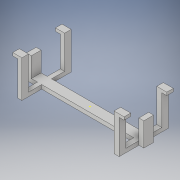
# Autodesk Inventor part: BatteryHanger
Saved by Autodesk Inventor 2018.2 (Build 222227000, 227)
## iProperties
Created: 2018-03-31
Part Number: BatteryHanger
Material: Generic
Document SubType Name: Modeling
Designer: MIABo
Density: 1 g/cm^3
Appearance: Default
Author: MIABo
Autodesk Inventor part; units mm, degrees
ref_plane "YZ Plane" through (0, 0, 0) normal (1, 0, 0) x (0, 1, 0)
ref_plane "XZ Plane" through (0, 0, 0) normal (0, 1, 0) x (-1, 0, 0)
ref_plane "XY Plane" through (0, 0, 0) normal (0, 0, 1) x (1, 0, 0)
sketch "Sketch1" plane through (0, 0, 0) normal (0, 1, 0) x (-1, 0, 0)
  line L0 (69.3801, 23.2918) -> (-69.3801, 23.2918)
  line L1 (-69.3801, 23.2918) -> (-69.3801, -23.2918)
  line L2 (-69.3801, -23.2918) -> (69.3801, -23.2918)
  line L3 (69.3801, -23.2918) -> (69.3801, 23.2918)
  line L4 (69.3801, 23.2918) -> (-69.3801, -23.2918) construction
  line L5 (-69.3801, 23.2918) -> (69.3801, -23.2918) construction
  line L6 (69.3801, -6.35) -> (-69.3801, -6.35)
  line L7 (-69.3801, -6.35) -> (-69.3801, 6.35)
  line L8 (-69.3801, 6.35) -> (69.3801, 6.35)
  line L9 (69.3801, 6.35) -> (69.3801, -6.35)
  line L10 (69.3801, -6.35) -> (-69.3801, 6.35) construction
  line L11 (-69.3801, -6.35) -> (69.3801, 6.35) construction
  line L12 (-62.7307, -31.75) -> (-69.3801, -31.75)
  line L13 (-69.3801, -31.75) -> (-69.3801, 31.75)
  line L14 (-69.3801, 31.75) -> (-62.7307, 31.75)
  line L15 (-62.7307, 31.75) -> (-62.7307, -31.75)
  line L16 (-62.7307, -31.75) -> (-69.3801, 31.75) construction
  line L17 (-69.3801, -31.75) -> (-62.7307, 31.75) construction
  line L18 (-69.3801, 0) -> (61.4807, 0)
  line L19 (61.4807, 0) -> (-69.3801, 0)
  line L20 (55.9943, 31.75) -> (55.9943, -31.75)
  line L21 (55.9943, -31.75) -> (61.4807, -31.75)
  line L22 (61.4807, -31.75) -> (61.4807, 31.75)
  line L23 (61.4807, 31.75) -> (55.9943, 31.75)
  line L24 (55.9943, 31.75) -> (61.4807, -31.75) construction
  line L25 (55.9943, -31.75) -> (61.4807, 31.75) construction
  point P0 (0, 0)
  point P1 (-66.0554, 0)
  point P2 (58.7375, 0)
  dimension "d0" = 138.7602
  dimension "d1" = 46.5836
  dimension "d2" = 12.7
  dimension "d3" = 130.8608
  constraints: 52 end point, 9 equal length, 9 midpoint, 5 perpendicular, 4 horizontal, 3 point on line
  measures "d0" distance of L2.end L1.end
  measures "d1" distance of L1.end L0.end
  measures "d2" distance of L6.end L7.end
  measures "d3" distance of L18.start L18.end
extrude "Extrusion1" add sketch "Sketch1" along normal blind 5.08 contours L22 L8 L20 L0 | L0 L20 L23 L22 | L3 L6 L22 L8 | L22 L18 L20 L8 | L15 L8 L1 L0 | L0 L13 L14 L15 | L20 L18 L15 L8 | L22 L6 L20 L18 | L22 L2 L20 L6 | L15 L18 L1 L8 | L20 L6 L15 L18 | L22 L21 L20 L2 | L15 L6 L1 L18 | L15 L2 L1 L6 | L15 L12 L13 L2
sketch "Sketch2" plane through (0, 5.08, 0) normal (0, 1, 0) x (1, 0, 0)
  point P0 (0, 0)
sketch "Sketch3" plane through (0, 0, 0) normal (0, -1, 0) x (1, 0, 0)
  line L0 (-69.3801, 6.35) -> (-61.4807, 6.35) projected
  line L1 (-69.3801, 6.35) -> (-75.7301, 6.35)
  line L2 (-75.7301, 6.35) -> (-75.7301, -6.35)
  line L3 (-75.7301, -6.35) -> (-69.3801, -6.35)
  line L4 (-69.3801, -6.35) -> (-69.3801, 6.35)
  line L5 (69.3801, 31.75) -> (69.3801, -31.75) projected
  line L6 (69.3801, 6.35) -> (75.7301, 6.35)
  line L7 (75.7301, 6.35) -> (75.7301, -6.35)
  line L8 (75.7301, -6.35) -> (69.3801, -6.35)
  line L9 (69.3801, -6.35) -> (69.3801, 6.35)
  point P0 (0, 0)
  dimension "d6" = 6.35
  dimension "d7" = 6.35
  constraints: 16 end point, 4 parallel, 3 point on line, 2 horizontal, 2 perpendicular
  measures "d6" distance of L3.end L2.end
  measures "d7" distance of L7.end L8.end
extrude "Extrusion2" add sketch "Sketch3" against normal blind 30.48
sketch "Sketch4" plane through (0, 5.08, 0) normal (0, 1, 0) x (1, 0, 0)
  line L0 (-69.3801, -23.2918) -> (69.3801, -23.2918)
  line L1 (69.3801, -23.2918) -> (69.3801, 23.2918)
  line L2 (69.3801, 23.2918) -> (-69.3801, 23.2918)
  line L3 (-69.3801, 23.2918) -> (-69.3801, -23.2918)
  line L4 (-69.3801, -23.2918) -> (69.3801, 23.2918) construction
  line L5 (69.3801, -23.2918) -> (-69.3801, 23.2918) construction
  line L6 (62.7307, 31.75) -> (62.7307, 6.35) projected
  line L7 (69.3801, 23.2918) -> (62.7307, 23.2918)
  line L8 (62.7307, 23.2918) -> (62.7307, 31.75)
  line L9 (62.7307, 31.75) -> (69.3801, 31.75)
  line L10 (69.3801, 31.75) -> (69.3801, 23.2918)
  line L11 (62.7307, -6.35) -> (62.7307, -31.75) projected
  line L12 (62.7307, -23.2918) -> (69.3801, -23.2918)
  line L13 (69.3801, -23.2918) -> (69.3801, -31.75)
  line L14 (69.3801, -31.75) -> (62.7307, -31.75)
  line L15 (62.7307, -31.75) -> (62.7307, -23.2918)
  line L16 (-61.4807, -31.75) -> (-55.9943, -31.75) projected
  line L17 (-61.4807, -6.35) -> (-61.4807, -31.75) projected
  line L18 (-55.9943, -31.75) -> (-61.4807, -31.75)
  line L19 (-61.4807, -31.75) -> (-61.4807, -23.2918)
  line L20 (-61.4807, -23.2918) -> (-55.9943, -23.2918)
  line L21 (-55.9943, -23.2918) -> (-55.9943, -31.75)
  line L22 (-61.4807, 31.75) -> (-61.4807, 6.35) projected
  line L23 (-55.9943, 31.75) -> (-61.4807, 31.75) projected
  line L24 (-61.4807, 23.2918) -> (-55.9943, 23.2918)
  line L25 (-55.9943, 23.2918) -> (-55.9943, 31.75)
  line L26 (-55.9943, 31.75) -> (-61.4807, 31.75)
  line L27 (-61.4807, 31.75) -> (-61.4807, 23.2918)
  point P0 (0, 0)
  dimension "d10" = 138.7602
  dimension "d11" = 46.5836
  constraints: 44 end point, 10 parallel, 7 point on line, 5 horizontal, 5 perpendicular, 2 midpoint
  measures "d10" distance of L2.end L1.end
  measures "d11" distance of L1.end L0.end
extrude "Extrusion3" add sketch "Sketch4" along normal blind 42.545 contours L0 L21 L16 L17 | L22 L23 L25 L2 | L0 L13 L14 L11 | L6 L9 L10 L2
sketch "Sketch5" plane through (69.3801, 0, -6.35) normal (1, 0, 0) x (0, 0, -1)
  line L0 (25.4, 47.625) -> (16.9418, 47.625) projected
  line L1 (25.4, 0) -> (25.4, 47.625) projected
  line L2 (16.9418, 47.625) -> (25.4, 47.625)
  line L3 (25.4, 47.625) -> (25.4, 43.815)
  line L4 (25.4, 43.815) -> (16.9418, 43.815)
  line L5 (16.9418, 43.815) -> (16.9418, 47.625)
  line L6 (-38.1, 0) -> (-38.1, 47.625) projected
  line L7 (-29.6418, 5.08) -> (-29.6418, 47.625) projected
  line L8 (-38.1, 47.625) -> (-29.6418, 47.625)
  line L9 (-29.6418, 47.625) -> (-29.6418, 43.815)
  line L10 (-29.6418, 43.815) -> (-38.1, 43.815)
  line L11 (-38.1, 43.815) -> (-38.1, 47.625)
  point P0 (-6.35, 0)
  dimension "d14" = 3.81
  constraints: 16 end point, 4 parallel, 2 horizontal, 2 perpendicular, 2 point on line
  measures "d14" distance of L2.end L3.end
extrude "Extrusion4" add sketch "Sketch5" along normal blind 6.35
sketch "Sketch6" plane through (-61.4807, 0, -31.75) normal (-1, 0, 0) x (0, 0, 1)
  line L0 (0, 0) -> (0, 47.625) projected
  line L1 (8.4582, 5.08) -> (8.4582, 47.625) projected
  line L2 (0, 47.625) -> (8.4582, 47.625)
  line L3 (8.4582, 47.625) -> (8.4582, 43.815)
  line L4 (8.4582, 43.815) -> (0, 43.815)
  line L5 (0, 43.815) -> (0, 47.625)
  line L6 (55.0418, 5.08) -> (55.0418, 47.625) projected
  line L7 (63.5, 0) -> (63.5, 47.625) projected
  line L8 (55.0418, 47.625) -> (63.5, 47.625)
  line L9 (63.5, 47.625) -> (63.5, 43.815)
  line L10 (63.5, 43.815) -> (55.0418, 43.815)
  line L11 (55.0418, 43.815) -> (55.0418, 47.625)
  point P0 (31.75, 0)
  dimension "d17" = 3.81
  constraints: 16 end point, 4 parallel, 3 point on line, 2 horizontal, 2 perpendicular
  measures "d17" distance of L2.end L3.end
extrude "Extrusion5" add sketch "Sketch6" along normal blind 6.35
body "Solid1"
